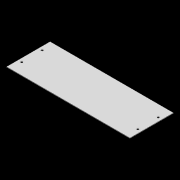
# Autodesk Inventor part: cannonplate
Saved by Autodesk Inventor 2022 (Build 260153000, 153)
## iProperties
Created: 2021-10-09
Part Number: cannonplate
Material: Generic
Document SubType Name: Modeling
Designer: timmy
Density: 1 g/cm^3
Appearance: Default
Author: timmy
Autodesk Inventor part; units mm, degrees
ref_plane "YZ Plane" through (0, 0, 0) normal (1, 0, 0) x (0, 1, 0)
ref_plane "XZ Plane" through (0, 0, 0) normal (0, 1, 0) x (-1, 0, 0)
ref_plane "XY Plane" through (0, 0, 0) normal (0, 0, 1) x (1, 0, 0)
sketch "Sketch1" plane through (0, 0, 0) normal (0, 1, 0) x (-1, 0, 0)
  line L0 (0, 0) -> (431.8, 0)
  line L1 (431.8, 0) -> (431.8, -152.4)
  line L2 (431.8, -152.4) -> (0, -152.4)
  line L3 (0, -152.4) -> (0, 0)
  dimension "d0" = 431.8
  dimension "d1" = 152.4
  constraints: 8 end point, 2 parallel, 1 horizontal, 1 perpendicular
  measures "d0" distance of L1.end L2.end
  measures "d1" distance of L0.end L1.end
extrude "Extrusion1" add sketch "Sketch1" along normal blind 1.5875
sketch "Sketch2" plane through (0, 1.5875, 0) normal (0, 1, 0) x (1, 0, 0)
  line L0 (0, 0) -> (0, 152.4) projected
  line L1 (0, 76.2) -> (-12.7, 76.2)
  line L2 (-431.8, 0) -> (0, 0) projected
  line L3 (-215.9, 0) -> (-215.9, 40.386)
  circle A0 centre (-12.7, 40.386) radius 3.175
  circle A1 centre (-419.1, 40.386) radius 3.175
  circle A2 centre (-12.7, 112.014) radius 3.175
  circle A3 centre (-419.1, 112.014) radius 3.175
  point P0 (-215.9, 112.014)
  dimension "d4" = 12.7
  dimension "d5" = 40.386
  dimension "d6" = 6.35
  constraints: 4 centre point, 4 end point, 4 symmetric about line, 2 midpoint, 1 horizontal, 1 vertical, 3 other
  measures "d4" distance of L1.start L1.end
  measures "d5" distance of L3.start L3.end
  measures "d6" diameter of A0
extrude "Extrusion2" cut sketch "Sketch2" against normal up to surface (1.5875 mm away)
body "Solid1"
